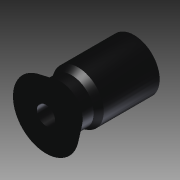
# Autodesk Inventor part: ZP08U_T_B
Saved by Autodesk Inventor 2011 SP1 (Build 150282100, 282)
## iProperties
Created: 2018-01-08
Part Number: ZP08U_T_B
Catalog Web Link: www.cadenas.de
Description: ZPT_2_8B_PAD-Vacuum Pad/Vertical Vacuum Entry With Buffer
Vendor: SMC
Document SubType Name: Modeling
Designer: psAdmin
Manufacturer: SMC
Mass: 0.395605 g
Surface Area: 4.61994 cm^2
Volume: 0.395605 cm^3
Density: 1 g/cm^3
Category: PARTsolutions
Company: SMC
Title: ZP08U
Author: Cadenas PARTsolutions
Comments: Vacuum Pad/Vertical Vacuum Entry With Buffer
PSOL_IDENT_0: {$CADENAS_DATA\23d-libs\smc_jp\vacuum_equipment\vacuum_pad\zp\zpt_b\zpt_2_8_b\parts\zpt_2_8_pad_b.pr
PSOL_IDENT_1: j},162 {VTYP=3D},{NB=ZP08U_T_B},{LINA=ZP08U},{NN=ZPT_2_8B_PAD},{DATE=12.07.2017 07:16:19},{GEOMDATE=
PSOL_IDENT_2: 28.02.2011 00:00:00},{VERSION=},{LINEID=60},{LINESUBID=-1},{WBVAR=}  {NB=ZP08U_T_B},{LINA=ZP08U},{KT=
PSOL_IDENT_3: DUMMY},{DIAMETER=8},{DIAMETERX=08},{PAD=(U) Flat},{PADX=U},{ORDER=ZP08U},{A=8.0},{B=9.0},{C=2.5},{Y=
PSOL_IDENT_4: 1.0},{DU=0.0},{EU=0.0}
NN: ZPT_2_8B_PAD
NT: Vacuum Pad/Vertical Vacuum Entry With Buffer
NB: ZP08U_T_B
NBSYN: $ORDER._T_B
LINA: ZP08U
DIAMETER: 8
PAD: (U) Flat
A: 8.0
B: 9.0
C: 2.5
Y: 1.0
DU: 0.0
EU: 0.0
SUPPLIER: SMC
ARTICLENO: ZP08U_T_B
BOMINFO: ZP08U
CREATOR: CADENAS GmbH
Autodesk Inventor part; units mm, degrees
sketch "Sketch_3" plane through (0, 0, 0) normal (0, 0, 1) x (1, 0, 0)
  line L0 (0, 0) -> (0, 12)
  line L1 (1.25, 12) -> (1.25, 0)
  line L2 (1.25, 0) -> (4.5, 0)
  line L3 (4.5, 0) -> (3, 2)
  line L4 (3, 2) -> (3, 3.5)
  line L5 (3, 3.5) -> (3.5, 4.37)
  line L6 (3.5, 4.37) -> (3.5, 12)
  line L7 (3.5, 12) -> (1.25, 12)
  constraints: 16 end point
revolve "Revolution1" add sketch "Sketch_3" angle 360 about axis through (0, 0, 0) along (0, -1, 0)
ref_plane "PAD_DUMMY_XY" through (0, 0, 0) normal (0, -1, 0) x (1, 0, 0)
ref_plane "PAD_DUMMY_YZ" through (0, 0, 0) normal (1, 0, 0) x (0, 0, 1)
ref_plane "PAD_DUMMY_ZX" through (0, 0, 0) normal (0, 0, 1) x (0, -1, 0)
ref_plane "pad_a_XY" through (0, 12, 0) normal (0, 1, 0) x (1, 0, 0)
ref_plane "pad_a_YZ" through (0, 12, 0) normal (1, 0, 0) x (0, 0, -1)
ref_plane "pad_a_ZX" through (0, 12, 0) normal (0, 0, -1) x (0, 1, 0)
body "Solid1"
